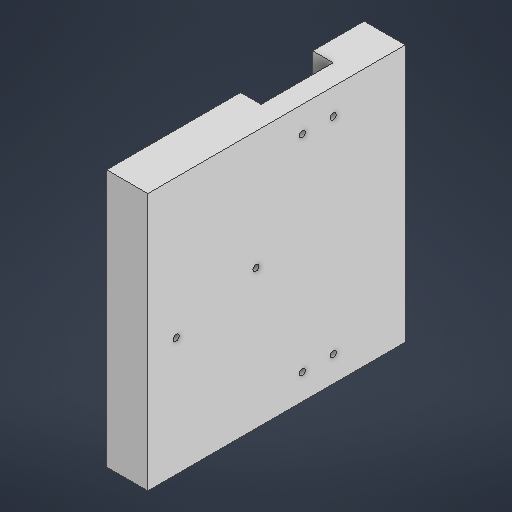
# Autodesk Inventor part: Suspension_Upright_V2_Topology_Baseline_V1
Saved by Autodesk Inventor 2026.1 (Build 301233000, 233)
## iProperties
Created: 2026-09-05
Part Number: Suspension_Upright_V2_Topology_Baseline_V1
Material: Generic
Document SubType Name: Modeling
Designer: share
Density: 1 g/cm^3
Appearance: Default
Author: share
Autodesk Inventor part; units mm, degrees
ref_plane "YZ Plane" through (0, 0, 0) normal (1, 0, 0) x (0, 1, 0)
ref_plane "XY Plane" through (0, 0, 0) normal (0, 0, 1) x (1, 0, 0)
sketch "Sketch1" plane through (0, 0, 0) normal (1, 0, 0) x (0, 1, 0)
  line L0 (0, 175) -> (0, -175) construction
  line L1 (-175, 0) -> (175, 0) construction
  line L2 (125, 125) -> (-125, 125)
  line L3 (-125, 125) -> (-125, -125)
  line L4 (-125, -125) -> (125, -125)
  line L5 (125, -125) -> (125, 125)
  point P0 (0, 0)
  dimension "d0" = 250
  dimension "d1" = 250
  constraints: 8 end point, 2 parallel, 1 horizontal, 1 perpendicular, 2 other
  measures "d0" distance between parallel lines of L4 L2
  measures "d1" distance between parallel lines of L3 L5
extrude "Main_Body" add sketch "Sketch1" along normal mid plane 40
sketch "Sketch4" plane through (-20, 0, 0) normal (-1, 0, 0) x (0, 0, 1)
  line L0 (-175, 0) -> (175, 0) construction
  line L1 (0, 175) -> (0, -175) construction
  line L2 (-55, 100) -> (-25, 100) construction
  line L3 (-55, -100) -> (-25, -100) construction
  line L4 (-40, 100) -> (-40, -100) construction
  line L5 (20, 10) -> (97.4597, -10) construction
  point P0 (0, 0)
  dimension "d10" = 30
  dimension "d12" = 40
  dimension "d13" = 200
  dimension "d21" = 80
  dimension "d22" = 60
  dimension "d23" = 10
  dimension "d24" = 10
  constraints: 8 end point, 2 horizontal, 2 midpoint, 2 symmetric about line, 1 parallel
  measures "d10" distance of L2.end L2.start
  measures "d12" distance between parallel lines of L1 L4
  measures "d13" distance between parallel lines of L3 L2
  measures "d21" distance of L5.start L5.end
  measures "d22" distance from line of L4 L5.start
  measures "d23" distance from line of L0 L5.start
  measures "d24" distance from line of L0 L5.end
hole "Hole1" at (-20, 100, -55) at (-20, 100, -25) at (-20, -100, -55) at (-20, -100, -25) at (-20, 10, 20) at (-20, -10, 97.4597) direction (1, 0, 0) diameter 6 end through all
sketch "Sketch5" plane through (-20, 0, 0) normal (-1, 0, 0) x (0, 0, 1)
  line L0 (125, 125) -> (-125, 125) projected
  line L1 (-75, 125) -> (-75, 85)
  line L2 (-75, 85) -> (-5, 85)
  line L3 (-5, 85) -> (-5, 125)
  line L4 (-40, 100) -> (-40, -100) construction
  line L5 (-175, 0) -> (175, 0) construction
  line L6 (-75, -125) -> (-75, -85)
  line L7 (-75, -85) -> (-5, -85)
  line L8 (-5, -85) -> (-5, -125)
  line L9 (-125, -125) -> (125, -125) projected
  circle A0 centre (-55, 100) radius 3 projected
  circle A1 centre (-25, 100) radius 3 projected
  circle A2 centre (-55, -100) radius 3 projected
  circle A3 centre (-25, -100) radius 3 projected
  point P0 (0, 0)
  dimension "d32" = 40
  dimension "d33" = 70
  constraints: 12 end point, 4 symmetric about line, 2 perpendicular, 2 point on line, 1 vertical, 1 other
  measures "d32" distance between parallel lines of L2 L0
  measures "d33" distance between parallel lines of L3 L1
extrude "L: Rock End Bracket Pocket" cut sketch "Sketch5" against normal up to surface (20 mm away)
sketch "Sketch8" plane through (20, 0, 0) normal (1, 0, 0) x (0, 0, -1)
  line L0 (40, 100) -> (40, -100) construction
  line L1 (-125, 125) -> (125, 125) projected
  line L2 (9.0545, 125) -> (9.0545, 85.102)
  line L3 (9.0545, 85.102) -> (70.9455, 85.102)
  line L4 (70.9455, 85.102) -> (70.9455, 125)
  line L5 (-175, 0) -> (175, 0) construction
  line L6 (9.0545, -125) -> (9.0545, -85.102)
  line L7 (9.0545, -85.102) -> (70.9455, -85.102)
  line L8 (70.9455, -85.102) -> (70.9455, -125)
  line L9 (-125, -125) -> (125, -125) projected
  circle A0 centre (25, 100) radius 3 projected
  circle A1 centre (55, 100) radius 3 projected
  circle A2 centre (25, -100) radius 3 projected
  circle A3 centre (55, -100) radius 3 projected
  point P0 (0, 0)
  dimension "d48" = 61.891
  dimension "d49" = 39.898
  constraints: 12 end point, 4 symmetric about line, 2 point on line, 1 horizontal, 1 perpendicular, 1 vertical, 1 other
  measures "d48" distance between parallel lines of L4 L2
  measures "d49" distance between parallel lines of L3 L1
extrude "R: Rod End Bracket Pocket" [suppressed]
sketch "Sketch9" plane through (-20, 0, 0) normal (-1, 0, 0) x (0, 0, 1)
  line L0 (-40, 100) -> (-40, -100) construction
  line L1 (-175, 0) -> (175, 0) construction
  circle A0 centre (-40, 0) radius 28.5745
  point P0 (0, 0)
  dimension "d52" = 57.149
  constraints: 1 centre point, 1 midpoint, 1 point on line
  measures "d52" diameter of A0
extrude "Axle Bore" [suppressed]
sketch "Sketch10" plane through (-20, 0, 0) normal (-1, 0, 0) x (0, 0, 1)
  circle A0 centre (-40, 0) radius 27.5 projected
  circle A1 centre (-40, 0) radius 37.9265
  point P0 (0, 0)
  dimension "d55" = 75.853
  constraints: 1 centre point, 1 coincident
  measures "d55" diameter of A1
extrude "Bearing Pocket 1" [suppressed]
sketch "Sketch11" plane through (20, 0, 0) normal (1, 0, 0) x (0, 0, -1)
  circle A0 centre (40, 0) radius 27.5 projected
  circle A1 centre (40, 0) radius 38.383
  point P0 (0, 0)
  dimension "d58" = 76.766
  constraints: 1 centre point, 1 coincident
  measures "d58" diameter of A1
extrude "Bearing Pocket 2" [suppressed]
ref_plane "Work Plane1" through (-20, 125, -125) normal (0, 1, 0) x (-1, 0, 0)
sketch "Sketch12" plane through (-20, 125, -125) normal (0, 1, 0) x (-1, 0, 0)
  line L0 (-20, -50) -> (-20, 300) construction
  line L1 (-48, 125) -> (8, 125) construction
  point P0 (-20, 125)
  point P1 (0, 85)
  point P2 (0, 85)
  point P3 (0, 85)
  point P4 (-20, 20.88)
  dimension "d61" = 64.12
  constraints: 1 point on line
  measures "d61" vertical distance of point (0, 85) point (-20, 20.88)
hole "Hole4" [suppressed]
sketch "Sketch13" plane through (20, 125, -125) normal (0, 0, -1) x (-1, 0, 0)
  line L0 (20, -300) -> (20, 50) construction
  line L1 (-8, -125) -> (48, -125) construction
  line L2 (40, -203.192) -> (0, -203.192)
  line L3 (0, -203.192) -> (0, -230.998)
  line L4 (0, -230.998) -> (40, -230.998)
  line L5 (40, -230.998) -> (40, -203.192)
  line L6 (0, -217.095) -> (40, -217.095) construction
  line L7 (0, -250) -> (0, 0) projected
  line L8 (40, 0) -> (40, -250) projected
  point P0 (20, -125)
  dimension "d69" = 92.095
  dimension "d70" = 27.806
  constraints: 10 end point, 2 collinear, 2 midpoint, 2 parallel, 1 horizontal, 1 perpendicular
  measures "d69" distance between parallel lines of L6 L1
  measures "d70" distance between parallel lines of L4 L2
extrude "Extrusion9" [suppressed]
equation "\"d32\" = Rod_End_Bracket_Slot_Height"
equation "\"d33\" = Rod_End_Bracket_Slot_Width"
equation "\"Rod_End_Bracket_Slot_Height\" = 40"
equation "\"Rod_End_Bracket_Slot_Width\" = 70"
body "Solid1"
